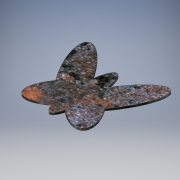
# Autodesk Inventor part: Butterfly
Saved by Autodesk Inventor 2019 (Build 230136000, 136)
## iProperties
Created: 2019-02-04
Part Number: Butterfly
Material: Generic
Document SubType Name: Modeling
Designer: mrhftc
Density: 1 g/cm^3
Appearance: Default
Author: mrhftc
Autodesk Inventor part; units mm, degrees
ref_plane "YZ Plane" through (0, 0, 0) normal (1, 0, 0) x (0, 1, 0)
ref_plane "XZ Plane" through (0, 0, 0) normal (0, 1, 0) x (-1, 0, 0)
ref_plane "Work Plane3" through (0, 2.54, 0) normal (0, 1, 0) x (1, 0, 0)
sketch "Sketch5" plane through (0, 2.54, 0) normal (0, 1, 0) x (1, 0, 0)
  ellipse E0 centre (201.451, 177.3473) end of major axis (229.2052, 221.1135) minor radius 16.0156 (208.013, 158.6416) -> (186.5008, 183.6371) ccw
  ellipse E1 centre (187.6899, 154.5313) end of major axis (215.633, 123.3862) minor radius 18.4642 (184.5561, 132.1117) -> (208.013, 158.6416) ccw
  ellipse E2 centre (176.9986, 162.7883) end of major axis (176.9986, 205.3655) minor radius 10.8982 (186.5008, 183.6371) -> (176.9986, 205.3655) ccw
  ellipse E3 centre (176.9986, 162.7883) end of major axis (176.9986, 205.3655) minor radius 10.8982 (176.9986, 120.211) -> (184.5561, 132.1117) ccw
  ellipse E4 centre (152.5463, 177.3473) end of major axis (124.7921, 221.1135) minor radius 16.0156 (167.4964, 183.6371) -> (145.9843, 158.6416) ccw
  ellipse E5 centre (166.3073, 154.5313) end of major axis (138.3642, 123.3862) minor radius 18.4642 (145.9843, 158.6416) -> (169.4411, 132.1117) ccw
  ellipse E6 centre (176.9986, 162.7883) end of major axis (176.9986, 205.3655) minor radius 10.8982 (176.9986, 205.3655) -> (167.4964, 183.6371) ccw
  ellipse E7 centre (176.9986, 162.7883) end of major axis (176.9986, 205.3655) minor radius 10.8982 (169.4411, 132.1117) -> (176.9986, 120.211) ccw
  ellipse E8 centre (166.3073, 154.5313) end of major axis (138.3642, 123.3862) minor radius 18.4642 (145.9843, 158.6416) -> (169.4411, 132.1117) ccw
  ellipse E9 centre (187.6899, 154.5313) end of major axis (215.633, 123.3862) minor radius 18.4642 (184.5561, 132.1117) -> (208.013, 158.6416) ccw
  point P0 (0, 0)
  constraints: 2 coincident, 40 other
extrude "Extrusion7" add sketch "Sketch5" along normal blind 2.54
body "Solid2"
